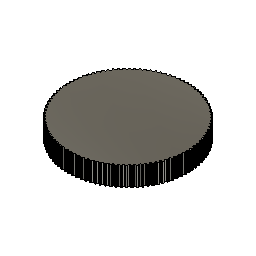
gear_98z (Autodesk Fusion 360 design; units mm, degrees)
Autodesk Fusion 360 part; units mm, degrees
sketch "Sketch1" plane through (0, 0, 0) normal (0, 0, 1) x (1, 0, 0) in component "gt2 pulley"
  circle A0 centre (0, 0) radius 31.1944 construction
  circle A1 centre (0, 0) radius 30.1904 construction
  line L0 (0, 0) -> (0, 31.1944) construction
  line L1 (0, 0) -> (0.9998, 31.1783) construction
  line L2 (0, 0) -> (1.4041, 31.1628) construction
  circle A2 centre (0, 0) radius 30.9404 construction
  arc A3 (0.3981, 30.805) -> (0.4776, 30.5058) centre (1.3927, 30.909) ccw
  circle A4 centre (0, 0) radius 30.7904 construction
  arc A5 (0.25, 30.9394) -> (0, 30.9404) centre (0, 0) ccw
  arc A6 (0.3981, 30.805) -> (0.25, 30.9394) centre (0.2489, 30.7894) ccw
  arc A7 (0.4776, 30.5058) -> (0.9676, 30.1749) centre (0.9854, 30.7296) ccw
  arc A8 (0, 30.9404) -> (-0.25, 30.9394) centre (0, 0) ccw
  arc A9 (-0.25, 30.9394) -> (-0.3981, 30.805) centre (-0.2489, 30.7894) ccw
  arc A10 (-0.4776, 30.5058) -> (-0.3981, 30.805) centre (-1.3927, 30.909) ccw
  arc A11 (-0.9678, 30.1749) -> (-0.4776, 30.5058) centre (-0.9854, 30.7296) ccw
  arc A12 (0.9676, 30.1749) -> (-0.9676, 30.1749) centre (0, 0) ccw
  point P0 (1.3927, 30.909)
  point P1 (0, 30.9404)
  dimension "d18" = 62.3887
  dimension "d19" = 1.837
  dimension "d22" = 1.004
  dimension "d24" = 0.75
  dimension "d26" = 1
  dimension "d27" = 0.15
  dimension "d28" = 0.15
  dimension "d47" = 0.555
  dimension "d52" = 3.812
  constraint coincident A0.centre A1.centre
  constraint coincident A0 L0.end
  constraint vertical L0
  constraint coincident A0 L1.end
  constraint coincident A0 L2.end
  constraint concentric A1 A2
  constraint coincident A1 A7.end
  constraint coincident L1 A7.end
  constraint coincident A2 P0
  constraint coincident L2 P0
  constraint coincident P0 A3.centre
  constraint coincident A2 P1
  constraint coincident L0 P1
  constraint concentric A2 A4
  constraint coincident P1 A5.end
  constraint coincident A4 A6.centre
  constraint coincident A3.start A6.start
  constraint tangent A3 A6
  constraint tangent A3 A7
  constraint symmetric L0 A7.end A12.end
  constraint symmetric L0 A3.start A9.end
  constraint symmetric L0 A3.end A10.start
  constraint symmetric L0 A3 A10
  constraint symmetric L0 A5.start A8.end
  constraint symmetric L0 P1 A5.end
  constraint symmetric L0 A5 A8
  constraint symmetric L0 A6 A9
  constraint symmetric L0 A7 A11
  constraint coincident A1 A11.start
  constraint tangent A1 A7
  constraint coincident L1 A7.centre
  measures "d18" diameter of A0
  measures "d19" angle of L0 L1
  measures "d22" distance of A0 A1
  measures "d24" distance of A1 A2
  measures "d26" radius of A3
  measures "d27" distance of A2 A4
  measures "d28" radius of A6
  measures "d47" radius of A7
extrude "Extrude1" add sketch "Sketch1" along normal blind 10 makes body 1
pattern_circular "C-Pattern1" count 98 over 360 about axis through (0, 0, 1.75) along (0, 0, 1) of bodies 1 makes body 2 at (-2.6849, 30.0707, 6.6667) makes body 3 at (-3.9674, 29.9286, 6.6667) makes body 4 at (-6.5082, 29.4805, 6.6667) makes body 5 at (-6.9275, 29.3848, 3.3333) makes body 6 at (-10.2247, 28.4062, 6.6667) makes body 7 at (-10.6283, 28.2577, 3.3333) makes body 8 at (-12.4169, 27.5187, 3.3333) makes body 9 at (-14.1545, 26.6666, 3.3333) makes body 10 at (-16.56, 25.2433, 6.6667) makes body 11 at (-18.6548, 23.7372, 6.6667) makes body 12 at (-18.9911, 23.4691, 3.3333) makes body 13 at (-21.3859, 21.3097, 6.6667) makes body 14 at (-22.8484, 19.7334, 6.6667) makes body 15 at (-23.1272, 19.406, 3.3333) makes body 16 at (-24.323, 17.8843, 3.3333) makes body 17 at (-25.8727, 15.5583, 6.6667) makes body 18 at (-26.8164, 13.8687, 6.6667) makes body 19 at (-27.6498, 12.1221, 6.6667) makes body 20 at (-28.5839, 9.717, 6.6667) makes body 21 at (-28.973, 8.4868, 6.6667) makes body 22 at (-29.5484, 6.1927, 6.6667) makes body 23 at (-29.8204, 4.7121, 6.6667) makes body 24 at (-30.061, 2.7918, 6.6667) makes body 25 at (-30.1414, 1.7196, 3.3333) makes body 26 at (-30.1896, -0.2151, 3.3333) makes body 27 at (-29.9692, -3.6474, 6.6667) makes body 28 at (-29.786, -4.9246, 6.6667) makes body 29 at (-29.2568, -7.4498, 6.6667) makes body 30 at (-28.7194, -9.309, 6.6667) makes body 31 at (-28.0639, -11.1299, 6.6667) makes body 32 at (-27.5627, -12.3189, 6.6667) makes body 33 at (-26.4103, -14.6273, 6.6667) makes body 34 at (-26.1992, -15.002, 3.3333) makes body 35 at (-24.3229, -17.8844, 6.6667) makes body 36 at (-23.1271, -19.4061, 6.6667) makes body 37 at (-22.8483, -19.7335, 3.3333) makes body 38 at (-20.6133, -22.0579, 6.6667) makes body 39 at (-20.1373, -22.4933, 3.3333) makes body 40 at (-18.6548, -23.7373, 3.3333) makes body 41 at (-17.0956, -24.8837, 3.3333) makes body 42 at (-14.1544, -26.6667, 6.6667) makes body 43 at (-13.1959, -27.1538, 6.6667) makes body 44 at (-11.2296, -28.0242, 6.6667) makes body 45 at (-9.4111, -28.6861, 6.6667) makes body 46 at (-6.9274, -29.3849, 6.6667) makes body 47 at (-5.0305, -29.7683, 6.6667) makes body 48 at (-3.3267, -30.0065, 6.6667) makes body 49 at (-1.1825, -30.1672, 6.6667) makes body 50 at (0.7528, -30.181, 6.6667) makes body 51 at (2.6849, -30.0707, 6.6667) makes body 52 at (3.9674, -29.9286, 6.6667) makes body 53 at (5.8767, -29.6129, 6.6667) makes body 54 at (6.9275, -29.3848, 6.6667) makes body 55 at (10.2247, -28.4062, 6.6667) makes body 56 at (12.0237, -27.6928, 6.6667) makes body 57 at (12.4169, -27.5187, 3.3333) makes body 58 at (14.1545, -26.6666, 3.3333) makes body 59 at (15.834, -25.7049, 3.3333) makes body 60 at (18.6548, -23.7372, 6.6667) makes body 61 at (18.9911, -23.4691, 3.3333) makes body 62 at (21.3859, -21.3097, 6.6667) makes body 63 at (22.8484, -19.7334, 6.6667) makes body 64 at (23.1272, -19.406, 3.3333) makes body 65 at (24.323, -17.8843, 3.3333) makes body 66 at (26.1993, -15.0019, 6.6667) makes body 67 at (26.4103, -14.6272, 3.3333) makes body 68 at (27.2932, -12.905, 3.3333) makes body 69 at (28.3697, -10.3257, 6.6667) makes body 70 at (28.973, -8.4868, 6.6667) makes body 71 at (29.2568, -7.4497, 6.6667) makes body 72 at (29.9143, -4.0738, 6.6667) makes body 73 at (30.061, -2.7918, 6.6667) makes body 74 at (30.1414, -1.7196, 3.3333) makes body 75 at (30.1896, 0.2151, 3.3333) makes body 76 at (29.9692, 3.6474, 6.6667) makes body 77 at (29.786, 4.9246, 6.6667) makes body 78 at (29.2568, 7.4498, 6.6667) makes body 79 at (28.7194, 9.309, 6.6667) makes body 80 at (28.5838, 9.7171, 3.3333) makes body 81 at (27.5627, 12.3189, 6.6667) makes body 82 at (26.5138, 14.4387, 3.3333) makes body 83 at (26.1992, 15.002, 3.3333) makes body 84 at (24.3229, 17.8844, 6.6667) makes body 85 at (23.2648, 19.2408, 6.6667) makes body 86 at (22.8483, 19.7335, 3.3333) makes body 87 at (20.6133, 22.0579, 6.6667) makes body 88 at (20.1373, 22.4933, 3.3333) makes body 89 at (18.6548, 23.7373, 3.3333) makes body 90 at (17.0956, 24.8837, 3.3333) makes body 91 at (14.1544, 26.6667, 6.6667) makes body 92 at (13.1959, 27.1538, 6.6667) makes body 93 at (11.429, 27.9434, 3.3333) makes body 94 at (10.2246, 28.4063, 3.3333) makes body 95 at (6.9274, 29.3849, 6.6667) makes body 96 at (5.0305, 29.7683, 6.6667) makes body 97 at (3.3267, 30.0065, 6.6667) makes body 98 at (2.6848, 30.0708, 3.3333)
sketch "Sketch2" plane through (0, 0, 10) normal (0, 0, 1) x (-1, 0, 0)
  arc A0 (-15.4634, -26.6456) -> (-15.4004, -26.8353) centre (-15.3257, -26.7052) ccw
  arc A1 (-15.4004, -26.8353) -> (-14.9646, -27.0807) centre (0, 0) ccw
  arc A2 (-14.9646, -27.0807) -> (-14.7697, -27.0363) centre (-14.892, -26.9495) ccw
  arc A3 (-14.5536, -26.8146) -> (-14.7697, -27.0363) centre (-13.9541, -27.615) ccw
  arc A4 (-13.9642, -26.7668) -> (-14.5536, -26.8146) centre (-14.2209, -27.2588) ccw
  arc A5 (-15.6505, -25.8171) -> (-13.9642, -26.7668) centre (0, 0) ccw
  arc A6 (-15.3858, -26.3459) -> (-15.6505, -25.8171) centre (-15.9382, -26.2917) ccw
  arc A7 (-15.4634, -26.6456) -> (-15.3858, -26.3459) centre (-16.381, -26.2482) ccw
  circle A8 centre (0, 0) radius 30.1904
  constraint coincident A1.centre A5.centre
extrude "Extrude2" add sketch "Sketch2" against normal blind 10 contours A5 A8 bodies 1 2 3 4 5 6 7 8 9 10 11 12 13 14 15 16 17 18 19 20 21 22 23 24 25 26 27 28 29 30 31 32 33 34 35 36 37 38 39 40 41 42 43 44 45 46 47 48 49 50 51 52 53 54 55 56 57 58 59 60 61 62 63 64 65 66 67 68 69 70 71 72 73 74 75 76 77 78 79 80 81 82 83 84 85 86 87 88 89 90 91 92 93 94 95 96 97 98
extrude "Extrude4" [suppressed] in component "gt2 pulley"
pattern_circular "C-Pattern7" [suppressed] in component "gt2 pulley"
extrude "Extrude3" [suppressed] in component "gt2 pulley"
pattern_circular "C-Pattern6" [suppressed] in component "gt2 pulley"
extrude "Extrude2'" [suppressed] in component "gt2 pulley"
pattern_circular "C-Pattern5" [suppressed] in component "gt2 pulley"
extrude "Extrude1'" [suppressed] in component "gt2 pulley"
pattern_circular "C-Pattern4" [suppressed] in component "gt2 pulley"
pattern_circular "C-Pattern3" [suppressed] in component "gt2 pulley"
pattern_circular "C-Pattern2" [suppressed] in component "gt2 pulley"
pattern_circular "C-Pattern1'" [suppressed] in component "gt2 pulley"
copy_body "Body->Comp1" [suppressed] in component "Component"
copy_body "Body->Comp2" [suppressed] in component "Component'"
copy_body "Body->Comp3" [suppressed] in component "Component''"
copy_body "Body->Comp4" [suppressed] in component "Component'''"
copy_body "Body->Comp5" [suppressed] in component "Component''''"
copy_body "Body->Comp6" [suppressed] in component "Component'''''"
copy_body "Body->Comp7" [suppressed] in component "Component''''''"
copy_body "Body->Comp8" [suppressed] in component "Component'''''''"
copy_body "Body->Comp9" [suppressed] in component "Component''''''''"
copy_body "Body->Comp10" [suppressed] in component "Component'''''''''"
copy_body "Body->Comp11" [suppressed] in component "Component''''''''''"
copy_body "Body->Comp12" [suppressed] in component "Component'''''''''''"
copy_body "Body->Comp13" [suppressed] in component "Component''''''''''''"
copy_body "Body->Comp14" [suppressed] in component "Component'''''''''''''"
copy_body "Body->Comp15" [suppressed] in component "Component''''''''''''''"
copy_body "Body->Comp16" [suppressed] in component "Component'''''''''''''''"
copy_body "Body->Comp17" [suppressed] in component "Component''''''''''''''''"
copy_body "Body->Comp18" [suppressed] in component "Component'''''''''''''''''"
copy_body "Body->Comp19" [suppressed] in component "Component''''''''''''''''''"
copy_body "Body->Comp20" [suppressed] in component "Component'''''''''''''''''''"
component "gt2 pulley" placed x (1, 0, 0) y (0, 1, 0) z (0, 0, 1) at (0, 0, 0)
equation "NumTeeth = 98" comment "min 20"
equation "ToothPitch = 2 mm"
equation "PullyDia = NumTeeth * ToothPitch / PI"
equation "ToothAng = ( ( 360 / NumTeeth ) * 1 deg )"
equation "TransOffsetAngle = ToothAng * 0.2"
equation "Sholulder_Radius = 0.15 mm"
equation "Root_Radius = 0.555 mm"
equation "TransRadius = 1 mm"
equation "ToolHeight = 0.75 mm"
equation "PLD = 0.254 mm"
equation "d18 = PullyDia"
equation "d19 = ToothAng / 2"
equation "d22 = PLD + ToolHeight"
equation "d24 = ToolHeight"
equation "d26 = TransRadius"
equation "d27 = Sholulder_Radius"
equation "d31 = NumTeeth"
equation "d33 = NumTeeth"
equation "d35 = NumTeeth"
equation "d37 = NumTeeth"
equation "d41 = NumTeeth"
equation "d45 = NumTeeth"
equation "d47 = Root_Radius"
equation "d50 = NumTeeth"
